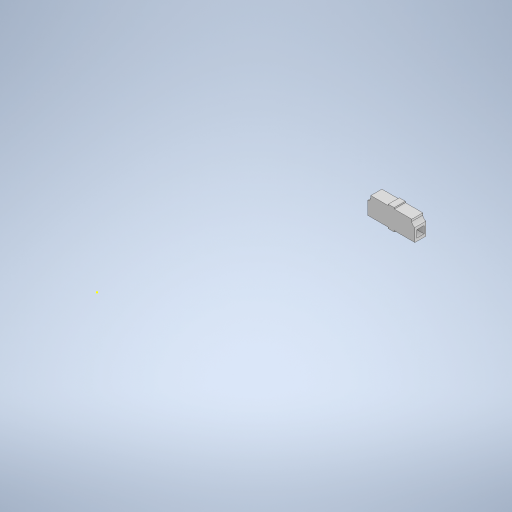
# Autodesk Inventor part: lc_lc_coupler_molex_1061251100_sd_scaled_3d
Saved by Autodesk Inventor 2024 (Build 280153000, 153)
## iProperties
Created: 2025-02-20
Part Number: lc_lc_coupler_molex_1061251100_sd_scaled_3d
Material: Generic
Document SubType Name: Modeling
Designer: phdgc
Density: 1 g/cm^3
Appearance: Default
Autodesk Inventor part; units mm, degrees
ref_plane "YZ Plane" through (0, 0, 0) normal (1, 0, 0) x (0, 1, 0)
ref_plane "XZ Plane" through (0, 0, 0) normal (0, 1, 0) x (-1, 0, 0)
ref_plane "XY Plane" through (0, 0, 0) normal (0, 0, 1) x (1, 0, 0)
sketch "Sketch1" plane through (0, 0, 0) normal (0, 0, 1) x (1, 0, 0)
  point P0 (0, 0)
sketch "0" plane through (0, 0, 0) normal (0, 0, 1) x (1, 0, 0)
  spline S0 degree 3 poles (174.458, 140.1191) (175.5599, 140.3052) (176.3666, 141.2594) (176.3666, 142.3769) knots 0 0 0 0 1 1 1 1
  line L0 (174.458, 140.1191) -> (175.5599, 140.3052) construction
  line L1 (175.5599, 140.3052) -> (176.3666, 141.2594) construction
  line L2 (176.3666, 141.2594) -> (176.3666, 142.3769) construction
  spline S1 degree 3 poles (201.7605, 142.3769) (201.7605, 141.2594) (202.5671, 140.3052) (203.6686, 140.1191) knots 0 0 0 0 1 1 1 1
  line L3 (201.7605, 142.3769) -> (201.7605, 141.2594) construction
  line L4 (201.7605, 141.2594) -> (202.5671, 140.3052) construction
  line L5 (202.5671, 140.3052) -> (203.6686, 140.1191) construction
  line L6 (187.2059, 144.3939) -> (189.0634, 144.3939)
  line L7 (187.2059, 144.3939) -> (187.2059, 142.2564)
  line L8 (190.9207, 144.3939) -> (190.9207, 142.9173)
  line L9 (203.6686, 132.066) -> (203.6686, 140.1191)
  line L10 (201.7605, 143.6175) -> (201.7605, 142.3769)
  line L11 (174.458, 132.066) -> (187.2059, 132.066)
  line L12 (176.3666, 143.6175) -> (187.2059, 143.6175)
  line L13 (174.458, 132.066) -> (174.458, 140.1191)
  line L14 (176.3666, 143.6175) -> (176.3666, 142.3769)
  line L15 (203.6686, 132.066) -> (190.9207, 132.066)
  line L16 (201.7605, 143.6175) -> (190.9207, 143.6175)
  line L17 (190.9207, 130.2365) -> (190.9207, 145.2514)
  line L18 (189.0634, 131.2896) -> (189.0634, 144.3939)
  line L19 (189.0634, 131.2896) -> (189.0634, 144.3939)
  line L20 (189.0634, 131.2896) -> (189.0634, 144.3939)
  line L21 (193.4909, 136.8872) -> (192.7376, 136.8872)
  line L22 (192.4867, 136.8872) -> (192.2352, 136.8872)
  line L23 (191.984, 136.8872) -> (190.4774, 136.8872)
  line L24 (190.226, 136.8872) -> (189.9748, 136.8872)
  line L25 (189.7238, 136.8872) -> (188.2172, 136.8872)
  line L26 (187.966, 136.8872) -> (187.7145, 136.8872)
  line L27 (187.4633, 136.8872) -> (185.9567, 136.8872)
  line L28 (185.7055, 136.8872) -> (185.4546, 136.8872)
  line L29 (185.2031, 136.8872) -> (184.4498, 136.8872)
  line L30 (190.9207, 131.2896) -> (189.0634, 131.2896)
  line L31 (187.2059, 131.2896) -> (187.2059, 133.4271)
  line L32 (187.2059, 131.2896) -> (189.0634, 131.2896)
  line L33 (190.9207, 131.2896) -> (190.9207, 132.7662)
  line L34 (190.9207, 144.3939) -> (189.0634, 144.3939)
  constraints: 58 end point, 7 point on line, 6 other
extrude "Extrusion1" add sketch "0" along normal blind 6.858
sketch "Sketch3" plane through (174.458, 132.066, 0) normal (-1, 0, 0) x (0, 0, 1)
  circle A0 centre (3.429, 4.0386) radius 0.625
  point P0 (0, -132.066)
  dimension "d2" = 1.25
  constraints: 1 centre point
  measures "d2" diameter of A0
extrude "Extrusion2" cut sketch "Sketch3" against normal through all
sketch "Sketch4" plane through (174.458, 132.066, 0) normal (-1, 0, 0) x (0, 0, 1)
  line L0 (1.194, 6.2736) -> (5.664, 6.2736)
  line L1 (5.664, 6.2736) -> (5.664, 1.8036)
  line L2 (5.664, 1.8036) -> (1.194, 1.8036)
  line L3 (1.194, 1.8036) -> (1.194, 6.2736)
  circle A0 centre (3.429, 4.0386) radius 0.625 projected
  line L4 (1.194, 6.2736) -> (5.664, 1.8036) construction
  line L5 (5.664, 6.2736) -> (1.194, 1.8036) construction
  point P0 (0, -132.066)
  dimension "d5" = 4.47
  dimension "d6" = 4.47
  constraints: 12 end point, 2 midpoint, 2 parallel, 1 horizontal, 1 perpendicular
  measures "d5" distance of L1.end L2.end
  measures "d6" distance of L0.end L1.end
extrude "Extrusion3" cut sketch "Sketch4" against normal blind 10
sketch "Sketch5" plane through (203.6686, 132.066, 0) normal (1, 0, 0) x (0, 0, -1)
  line L0 (-5.664, 1.8036) -> (-1.194, 1.8036) projected
  line L1 (-5.664, 6.2736) -> (-1.194, 6.2736)
  line L2 (-1.194, 6.2736) -> (-1.194, 1.8036)
  line L3 (-1.194, 1.8036) -> (-5.664, 1.8036)
  line L4 (-5.664, 1.8036) -> (-5.664, 6.2736)
  circle A0 centre (-3.429, 4.0386) radius 0.625 projected
  line L5 (-5.664, 6.2736) -> (-1.194, 1.8036) construction
  line L6 (-1.194, 6.2736) -> (-5.664, 1.8036) construction
  point P0 (0, -132.066)
  constraints: 12 end point, 2 midpoint, 2 parallel, 1 horizontal, 1 perpendicular
extrude "Extrusion4" cut sketch "Sketch5" against normal blind 10
body "Solid1"
